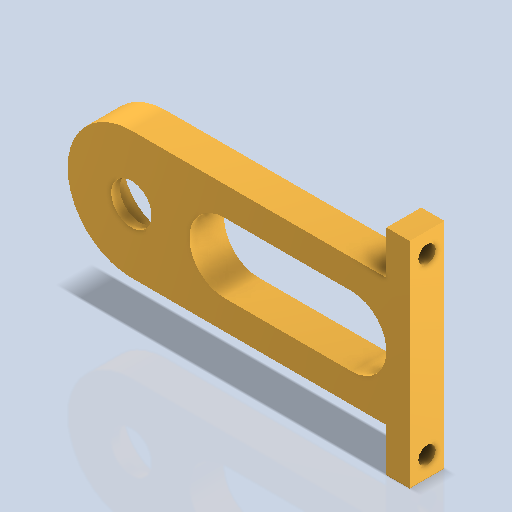
# Autodesk Inventor part: 1
Saved by Autodesk Inventor 2024.2 (Build 282272000, 272)
## iProperties
Created: 2024-05-04
Part Number: 1
Material: Messing, weicher Gelbton
Document SubType Name: Modeling
Designer: Fabri
Density: 8.47 g/cm^3
Appearance: Messing - satiniert
Author: Fabri
Autodesk Inventor part; units mm, degrees
ref_plane "YZ Plane" through (0, 0, 0) normal (1, 0, 0) x (0, 1, 0)
ref_plane "XZ Plane" through (0, 0, 0) normal (0, 1, 0) x (-1, 0, 0)
ref_plane "XY Plane" through (0, 0, 0) normal (0, 0, 1) x (1, 0, 0)
sketch "Skizze1" plane through (0, 0, 0) normal (0, 1, 0) x (-1, 0, 0)
  line L0 (0, 0) -> (0, 74)
  line L1 (0, 74) -> (16, 74)
  line L2 (16, 74) -> (16, 44)
  line L3 (16, 44) -> (192, 44)
  arc A0 (192, -44) -> (192, 44) centre (192, 0) ccw
  line L4 (192, -44) -> (16, -44)
  line L5 (16, -44) -> (16, -74)
  line L6 (16, -74) -> (0, -74)
  line L7 (0, -74) -> (0, 0)
  line L8 (0, 0) -> (236, 0) construction
  dimension "d0" = 192
  dimension "d1" = 16
  dimension "d2" = 30
  dimension "d3" = 44
  constraints: 18 end point, 5 perpendicular, 3 point on circle, 3 point on line, 1 centre point, 1 horizontal, 1 parallel, 1 symmetric about line, 1 tangent, 1 vertical, 1 other
  measures "d0" distance from line of L7 A0.centre
  measures "d1" distance between parallel lines of L7 L5
  measures "d2" distance between parallel lines of L1 L3
  measures "d3" radius of A0
extrude "Extrusion1" add sketch "Skizze1" along normal blind 24
sketch "Skizze2" plane through (0, 24, 0) normal (0, 1, 0) x (1, 0, 0)
  arc A0 (-192, 44) -> (-192, -44) centre (-192, 0) ccw projected
  point P0 (0, 0)
  constraints: 1 coincident
hole "Bohrung1" at (-192, 24, 0) direction (0, -1, 0) diameter 60 depth 18
sketch "Skizze3" plane through (-192, 6, 0) normal (0, 1, 0) x (1, 0, 0)
  circle A0 centre (0, 0) radius 30 projected
  point P0 (192, 0)
  constraints: 1 coincident
hole "Bohrung2" at (-192, 6, 0) direction (0, -1, 0) diameter 28 depth 6
sketch "Skizze4" plane through (0, 24, 0) normal (0, 1, 0) x (1, 0, 0)
  line L0 (-40, 0) -> (-128, 0) construction
  line L1 (-40, 24) -> (-128, 24)
  line L2 (-128, -24) -> (-40, -24)
  arc A0 (-40, -24) -> (-40, 24) centre (-40, 0) ccw
  arc A1 (-128, 24) -> (-128, -24) centre (-128, 0) ccw
  line L3 (0, -74) -> (0, 74) projected
  line L4 (-16, -44) -> (-16, -74) projected
  point P0 (0, 0)
  point P1 (-84, 0)
  point P2 (0, 0)
  point P3 (0, 0)
  dimension "d20" = 88
  dimension "d21" = 48
  dimension "d22" = 24
  constraints: 8 end point, 4 point on circle, 4 tangent, 3 midpoint, 2 centre point, 2 horizontal alignment, 1 parallel
  measures "d20" distance of L0.start L0.end
  measures "d21" distance between parallel lines of L1 L2
  measures "d22" distance from line of L4 L0.start
extrude "Extrusion2" cut sketch "Skizze4" against normal up to surface (24 mm away)
sketch "Skizze5" plane through (-16, 0, -74) normal (-1, 0, 0) x (0, 0, 1)
  line L0 (148, 0) -> (148, 24) projected
  line L1 (0, 0) -> (0, 24) projected
  point P0 (74, 0)
  point P1 (14, 12)
  point P2 (134, 12)
  point P3 (148, 12)
  point P4 (0, 12)
  dimension "d32" = 120
  dimension "d33" = 60
  constraints: 2 horizontal alignment, 2 midpoint
  measures "d32" distance of point (14, 12) point (134, 12)
  measures "d33" horizontal distance of point (74, 0) point (134, 12)
hole "Bohrung3" at (-16, 12, -60) at (-16, 12, 60) direction (1, 0, 0) diameter 12 depth 16
